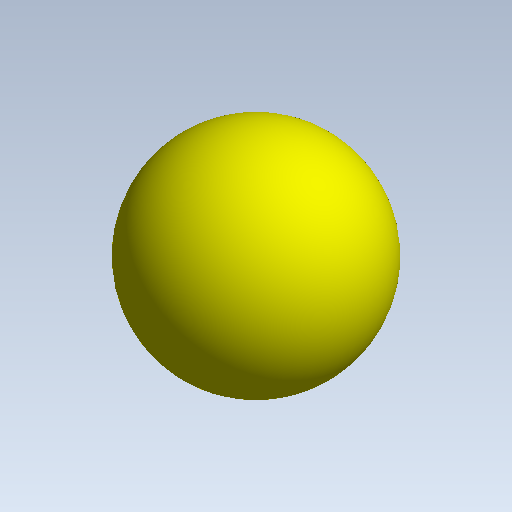
# Autodesk Inventor part: W 637/5 X-2Z_PART3
Saved by Autodesk Inventor 2021 (Build 250183000, 183)
## iProperties
Part Number: W 637/5 X-2Z_PART3
Material: Allgemein
Catalog Web Link: www.cadenas.de
Description: -Deep groove ball bearings
Vendor: SKF
Document SubType Name: Modeling
Designer: partserver
Manufacturer: SKF
Mass: 0.000904779 g
Surface Area: 0.0452389 cm^2
Volume: 0.000904779 cm^3
Density: 1 g/cm^3
Appearance: PSOLRGB-192-192-192
Category: PARTsolutions
Company: SKF
PSOL_IDENT_0: {$CADENAS_DATA\23d-libs\skf\bearings_units_and_housings\ball_bearings\deep_groove_ball_bearings\bb1_
PSOL_IDENT_1: 001_101.prj},203 {VTYP=3D},{NB=W 637/5 X-2Z_PART3},{LINA=W 637/5 X-2Z_PART3},{NN=BB1_001_101_PART3},
PSOL_IDENT_2: {NOPRJ=TRUE},{DATE=19.12.2019 14:34:47},{GEOMDATE=18.12.2019 13:53:11},{VERSION=},{LINEID=20320},{WB
PSOL_IDENT_3: VAR=},{WBNUMERIC=}  {NB=W 637/5 X-2Z_PART3},{LINA=W 637/5 X-2Z_PART3},{KT=DUMMY},{PRODUCTID=},{DESIG
PSOL_IDENT_4: NATION=W 637/5 X-2Z},{DD=5.000},{D=9.000},{B=3.000},{C=0.000},{DD1=6.00},{DD2=0.00},{D1=0.00},{D2=8.
PSOL_IDENT_5: 40},{D3=0.000},{D4=0.000},{HH=MIN},{BB=0.000},{FF=0.00},{R0MAX=MIN},{R0=MIN},{R12=0.15},{PITCH=6.90}
PSOL_IDENT_6: ,{DW=1.200},{DDAMIN=5.900},{DDAMAX=5.900},{DDBMIN=MIN},{DDBMAX=MIN},{DBMIN=MIN},{DAMAX=8.400},{BBAMI
PSOL_IDENT_7: N=MIN},{CAMAX=MIN},{RAMAX=0.150},{LOAD1=0.247},{LOAD2=0.085},{LOAD3=0.004},{SPEED1=130000},{SPEED2=6
PSOL_IDENT_8: 7000},{KR=0.020},{F0=7.600},{Z=8},{II=1},{MASS=0.001},{BEARING=W 637/5 X-2Z},{RING=},{HELP=0.648},{H
PSOL_IDENT_9: ELP2=0.300},{DD1ALG=3.000},{YALG=3.000},{PITCH1=6.900},{DW1=1.200},{YALG1=3.852},{HALG1=0.648},{SH=3
PSOL_IDENT_10: .000},{CU=0.360},{DESIGN=dgbbw2z},{HALG=0.5},{B1=0},{SHIELDHELP=2}
NB: W 637/5 X-2Z_PART3
NT: Deep groove ball bearings
NBSYN: $DESIGNATION._PART3
LINA: W 637/5 X-2Z_PART3
CATALOG: SKF
SUPPLIER: SKF
ARTICLENO: W 637/5 X-2Z_PART3
BOMINFO: W 637/5 X-2Z_PART3
CREATOR: CADENAS GmbH
Title: W 637/5 X-2Z_PART3
Author: Cadenas PARTsolutions
Comments: Deep groove ball bearings
Autodesk Inventor part; units mm, degrees
ref_plane "YZ Plane" through (0, 0, 0) normal (1, 0, 0) x (0, 1, 0)
ref_plane "XZ Plane" through (0, 0, 0) normal (0, 1, 0) x (-1, 0, 0)
ref_plane "XY Plane" through (0, 0, 0) normal (0, 0, 1) x (1, 0, 0)
sketch "Sketch_6" plane through (0, 0, 0) normal (0, 0, 1) x (1, 0, 0)
  line L0 (2.1, 3.45) -> (0.9, 3.45)
  arc A0 (2.1, 3.45) -> (0.9, 3.45) centre (1.5, 3.45) ccw
  line L1 (2.1, 3.45) -> (0.9, 3.45)
  dimension "d0" = 360
  constraints: 4 end point, 2 point on circle, 1 centre point
revolve "Revolution1" add sketch "Sketch_6" angle 360 about axis through (2.1, 3.45, 0) along (1, 0, 0)
body "Solid1"
